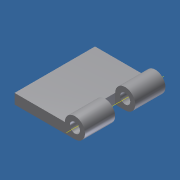
# Autodesk Inventor part: hinge two prong
Saved by Autodesk Inventor 2012 (Build 160160000, 160)
## iProperties
Created: 2012-02-06
Part Number: hinge two prong
Material: Default
Document SubType Name: Modeling
Designer: Allison Garza
Density: 1 g/cm^3
Author: Allison Garza
Autodesk Inventor part; units mm, degrees
ref_plane "YZ Plane" through (0, 0, 0) normal (1, 0, 0) x (0, 1, 0)
ref_plane "XZ Plane" through (0, 0, 0) normal (0, 1, 0) x (-1, 0, 0)
ref_plane "XY Plane" through (0, 0, 0) normal (0, 0, 1) x (1, 0, 0)
sketch "Sketch1" plane through (0, 0, 0) normal (0, 0, 1) x (1, 0, 0)
  circle A0 centre (0, 0) radius 3.175
  circle A1 centre (0, 0) radius 1.5875
  line L0 (0, -3.175) -> (-19.05, -3.175)
  line L1 (-19.05, -3.175) -> (-19.05, 0)
  line L2 (-19.05, 0) -> (-1.5875, 0)
  line L3 (0, -1.5875) -> (0, -3.175)
  dimension "d0" = 6.35
  dimension "d1" = 3.175
  dimension "d2" = 19.05
  dimension "d3" = 3.175
  constraints: 8 end point, 3 coincident, 2 parallel, 2 point on circle, 1 centre point, 1 horizontal, 1 perpendicular, 1 vertical alignment, 2 other
  measures "d1" diameter of A1
  measures "d2" distance of L0.start L0.end
  measures "d3" distance of L0.end L1.end
extrude "Extrusion1" add sketch "Sketch1" along normal blind 25.4 contours L3 A1 L2 A0 | L0 L1 L2 A0 | A0 L2 A1 L3
sketch "Sketch2" plane through (-19.05, -3.175, 0) normal (0, -1, 0) x (1, 0, 0)
  line L0 (15.875, 15.875) -> (22.225, 15.875)
  line L1 (22.225, 15.875) -> (22.225, 9.525)
  line L2 (22.225, 9.525) -> (15.875, 9.525)
  line L3 (15.875, 9.525) -> (15.875, 15.875)
  line L4 (15.875, 25.4) -> (22.225, 25.4) projected
  point P0 (19.05, 0)
  dimension "d6" = 6.35
  dimension "d7" = 3.175
  dimension "d8" = 6.35
  dimension "d9" = 9.525
  constraints: 8 end point, 2 parallel, 1 horizontal, 1 perpendicular
  measures "d6" distance of L0.start L0.end
  measures "d7" horizontal distance of point (19.05, 0) L2.end
  measures "d8" distance of L0.end L1.end
  measures "d9" distance from line of L4 L0.end
extrude "Extrusion2" cut sketch "Sketch2" against normal blind 25.4
body "Solid1"
